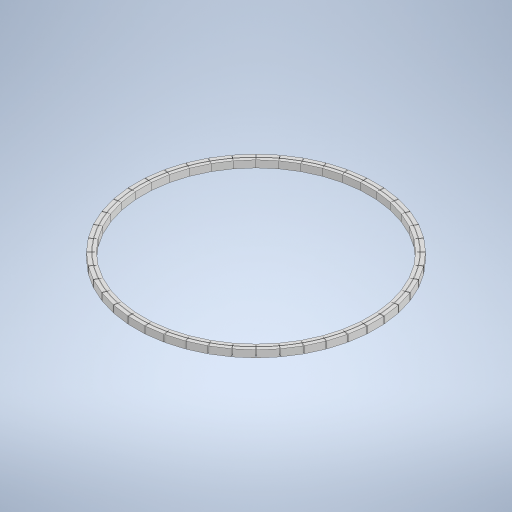
# Autodesk Inventor part: 柱-1 磚-1
Saved by Autodesk Inventor 2024 (Build 280153000, 153)
## iProperties
Created: 2024-05-18
Part Number: 柱-1 磚-1
Material: 一般
Document SubType Name: Modeling
Designer: User
Density: 1 g/cm^3
Appearance: 預設
Author: User
Autodesk Inventor part; units mm, degrees
ref_plane "YZ Plane" through (0, 0, 0) normal (1, 0, 0) x (0, 1, 0)
ref_plane "XZ Plane" through (0, 0, 0) normal (0, 1, 0) x (-1, 0, 0)
ref_plane "XY Plane" through (0, 0, 0) normal (0, 0, 1) x (1, 0, 0)
sketch "草圖1" plane through (0, 0, 0) normal (0, 1, 0) x (-1, 0, 0)
  circle A0 centre (0, 0) radius 25
  line L0 (24.25, 1.75) -> (25.75, 1.75)
  line L1 (25.75, 1.75) -> (25.75, -1.75)
  line L2 (25.75, -1.75) -> (24.25, -1.75)
  line L3 (24.25, -1.75) -> (24.25, 1.75)
  line L4 (24.25, 1.75) -> (25.75, -1.75) construction
  line L5 (25.75, 1.75) -> (24.25, -1.75) construction
  line L6 (25.2389, 5.3968) -> (25.737, 1.9324)
  line L7 (25.737, 1.9324) -> (24.2522, 1.7189)
  line L8 (24.2522, 1.7189) -> (23.7541, 5.1833)
  line L9 (23.7541, 5.1833) -> (25.2389, 5.3968)
  line L10 (24.2139, 8.9337) -> (25.2, 5.5755)
  line L11 (25.2, 5.5755) -> (23.7607, 5.1529)
  line L12 (23.7607, 5.1529) -> (22.7747, 8.5111)
  line L13 (22.7747, 8.5111) -> (24.2139, 8.9337)
  line L14 (22.696, 12.2888) -> (24.15, 9.1051)
  line L15 (24.15, 9.1051) -> (22.7856, 8.482)
  line L16 (22.7856, 8.482) -> (21.3316, 11.6657)
  line L17 (21.3316, 11.6657) -> (22.696, 12.2888)
  line L18 (20.7162, 15.3937) -> (22.6084, 12.4493)
  line L19 (22.6084, 12.4493) -> (21.3465, 11.6383)
  line L20 (21.3465, 11.6383) -> (19.4543, 14.5827)
  line L21 (19.4543, 14.5827) -> (20.7162, 15.3937)
  line L22 (18.3145, 18.1852) -> (20.6066, 15.5401)
  line L23 (20.6066, 15.5401) -> (19.4729, 14.5578)
  line L24 (19.4729, 14.5578) -> (17.1809, 17.2029)
  line L25 (17.1809, 17.2029) -> (18.3145, 18.1852)
  line L26 (15.5401, 20.6066) -> (18.1852, 18.3145)
  line L27 (18.1852, 18.3145) -> (17.2029, 17.1809)
  line L28 (17.2029, 17.1809) -> (14.5578, 19.4729)
  line L29 (14.5578, 19.4729) -> (15.5401, 20.6066)
  line L30 (12.4493, 22.6084) -> (15.3937, 20.7162)
  line L31 (15.3937, 20.7162) -> (14.5827, 19.4543)
  line L32 (14.5827, 19.4543) -> (11.6383, 21.3465)
  line L33 (11.6383, 21.3465) -> (12.4493, 22.6084)
  line L34 (9.1051, 24.15) -> (12.2888, 22.696)
  line L35 (12.2888, 22.696) -> (11.6657, 21.3316)
  line L36 (11.6657, 21.3316) -> (8.482, 22.7856)
  line L37 (8.482, 22.7856) -> (9.1051, 24.15)
  line L38 (5.5755, 25.2) -> (8.9337, 24.2139)
  line L39 (8.9337, 24.2139) -> (8.5111, 22.7747)
  line L40 (8.5111, 22.7747) -> (5.1529, 23.7607)
  line L41 (5.1529, 23.7607) -> (5.5755, 25.2)
  line L42 (1.9324, 25.737) -> (5.3968, 25.2389)
  line L43 (5.3968, 25.2389) -> (5.1833, 23.7541)
  line L44 (5.1833, 23.7541) -> (1.7189, 24.2522)
  line L45 (1.7189, 24.2522) -> (1.9324, 25.737)
  line L46 (-1.75, 25.75) -> (1.75, 25.75)
  line L47 (1.75, 25.75) -> (1.75, 24.25)
  line L48 (1.75, 24.25) -> (-1.75, 24.25)
  line L49 (-1.75, 24.25) -> (-1.75, 25.75)
  line L50 (-5.3968, 25.2389) -> (-1.9324, 25.737)
  line L51 (-1.9324, 25.737) -> (-1.7189, 24.2522)
  line L52 (-1.7189, 24.2522) -> (-5.1833, 23.7541)
  line L53 (-5.1833, 23.7541) -> (-5.3968, 25.2389)
  line L54 (-8.9337, 24.2139) -> (-5.5755, 25.2)
  line L55 (-5.5755, 25.2) -> (-5.1529, 23.7607)
  line L56 (-5.1529, 23.7607) -> (-8.5111, 22.7747)
  line L57 (-8.5111, 22.7747) -> (-8.9337, 24.2139)
  line L58 (-12.2888, 22.696) -> (-9.1051, 24.15)
  line L59 (-9.1051, 24.15) -> (-8.482, 22.7856)
  line L60 (-8.482, 22.7856) -> (-11.6657, 21.3316)
  line L61 (-11.6657, 21.3316) -> (-12.2888, 22.696)
  line L62 (-15.3937, 20.7162) -> (-12.4493, 22.6084)
  line L63 (-12.4493, 22.6084) -> (-11.6383, 21.3465)
  line L64 (-11.6383, 21.3465) -> (-14.5827, 19.4543)
  line L65 (-14.5827, 19.4543) -> (-15.3937, 20.7162)
  line L66 (-18.1852, 18.3145) -> (-15.5401, 20.6066)
  line L67 (-15.5401, 20.6066) -> (-14.5578, 19.4729)
  line L68 (-14.5578, 19.4729) -> (-17.2029, 17.1809)
  line L69 (-17.2029, 17.1809) -> (-18.1852, 18.3145)
  line L70 (-20.6066, 15.5401) -> (-18.3145, 18.1852)
  line L71 (-18.3145, 18.1852) -> (-17.1809, 17.2029)
  line L72 (-17.1809, 17.2029) -> (-19.4729, 14.5578)
  line L73 (-19.4729, 14.5578) -> (-20.6066, 15.5401)
  line L74 (-22.6084, 12.4493) -> (-20.7162, 15.3937)
  line L75 (-20.7162, 15.3937) -> (-19.4543, 14.5827)
  line L76 (-19.4543, 14.5827) -> (-21.3465, 11.6383)
  line L77 (-21.3465, 11.6383) -> (-22.6084, 12.4493)
  line L78 (-24.15, 9.1051) -> (-22.696, 12.2888)
  line L79 (-22.696, 12.2888) -> (-21.3316, 11.6657)
  line L80 (-21.3316, 11.6657) -> (-22.7856, 8.482)
  line L81 (-22.7856, 8.482) -> (-24.15, 9.1051)
  line L82 (-25.2, 5.5755) -> (-24.2139, 8.9337)
  line L83 (-24.2139, 8.9337) -> (-22.7747, 8.5111)
  line L84 (-22.7747, 8.5111) -> (-23.7607, 5.1529)
  line L85 (-23.7607, 5.1529) -> (-25.2, 5.5755)
  line L86 (-25.737, 1.9324) -> (-25.2389, 5.3968)
  line L87 (-25.2389, 5.3968) -> (-23.7541, 5.1833)
  line L88 (-23.7541, 5.1833) -> (-24.2522, 1.7189)
  line L89 (-24.2522, 1.7189) -> (-25.737, 1.9324)
  line L90 (-25.75, -1.75) -> (-25.75, 1.75)
  line L91 (-25.75, 1.75) -> (-24.25, 1.75)
  line L92 (-24.25, 1.75) -> (-24.25, -1.75)
  line L93 (-24.25, -1.75) -> (-25.75, -1.75)
  line L94 (-25.2389, -5.3968) -> (-25.737, -1.9324)
  line L95 (-25.737, -1.9324) -> (-24.2522, -1.7189)
  line L96 (-24.2522, -1.7189) -> (-23.7541, -5.1833)
  line L97 (-23.7541, -5.1833) -> (-25.2389, -5.3968)
  line L98 (-24.2139, -8.9337) -> (-25.2, -5.5755)
  line L99 (-25.2, -5.5755) -> (-23.7607, -5.1529)
  line L100 (-23.7607, -5.1529) -> (-22.7747, -8.5111)
  line L101 (-22.7747, -8.5111) -> (-24.2139, -8.9337)
  line L102 (-22.696, -12.2888) -> (-24.15, -9.1051)
  line L103 (-24.15, -9.1051) -> (-22.7856, -8.482)
  line L104 (-22.7856, -8.482) -> (-21.3316, -11.6657)
  line L105 (-21.3316, -11.6657) -> (-22.696, -12.2888)
  line L106 (-20.7162, -15.3937) -> (-22.6084, -12.4493)
  line L107 (-22.6084, -12.4493) -> (-21.3465, -11.6383)
  line L108 (-21.3465, -11.6383) -> (-19.4543, -14.5827)
  line L109 (-19.4543, -14.5827) -> (-20.7162, -15.3937)
  line L110 (-18.3145, -18.1852) -> (-20.6066, -15.5401)
  line L111 (-20.6066, -15.5401) -> (-19.4729, -14.5578)
  line L112 (-19.4729, -14.5578) -> (-17.1809, -17.2029)
  line L113 (-17.1809, -17.2029) -> (-18.3145, -18.1852)
  line L114 (-15.5401, -20.6066) -> (-18.1852, -18.3145)
  line L115 (-18.1852, -18.3145) -> (-17.2029, -17.1809)
  line L116 (-17.2029, -17.1809) -> (-14.5578, -19.4729)
  line L117 (-14.5578, -19.4729) -> (-15.5401, -20.6066)
  line L118 (-12.4493, -22.6084) -> (-15.3937, -20.7162)
  line L119 (-15.3937, -20.7162) -> (-14.5827, -19.4543)
  line L120 (-14.5827, -19.4543) -> (-11.6383, -21.3465)
  line L121 (-11.6383, -21.3465) -> (-12.4493, -22.6084)
  line L122 (-9.1051, -24.15) -> (-12.2888, -22.696)
  line L123 (-12.2888, -22.696) -> (-11.6657, -21.3316)
  line L124 (-11.6657, -21.3316) -> (-8.482, -22.7856)
  line L125 (-8.482, -22.7856) -> (-9.1051, -24.15)
  line L126 (-5.5755, -25.2) -> (-8.9337, -24.2139)
  line L127 (-8.9337, -24.2139) -> (-8.5111, -22.7747)
  line L128 (-8.5111, -22.7747) -> (-5.1529, -23.7607)
  line L129 (-5.1529, -23.7607) -> (-5.5755, -25.2)
  line L130 (-1.9324, -25.737) -> (-5.3968, -25.2389)
  line L131 (-5.3968, -25.2389) -> (-5.1833, -23.7541)
  line L132 (-5.1833, -23.7541) -> (-1.7189, -24.2522)
  line L133 (-1.7189, -24.2522) -> (-1.9324, -25.737)
  line L134 (1.75, -25.75) -> (-1.75, -25.75)
  line L135 (-1.75, -25.75) -> (-1.75, -24.25)
  line L136 (-1.75, -24.25) -> (1.75, -24.25)
  line L137 (1.75, -24.25) -> (1.75, -25.75)
  line L138 (5.3968, -25.2389) -> (1.9324, -25.737)
  line L139 (1.9324, -25.737) -> (1.7189, -24.2522)
  line L140 (1.7189, -24.2522) -> (5.1833, -23.7541)
  line L141 (5.1833, -23.7541) -> (5.3968, -25.2389)
  line L142 (8.9337, -24.2139) -> (5.5755, -25.2)
  line L143 (5.5755, -25.2) -> (5.1529, -23.7607)
  line L144 (5.1529, -23.7607) -> (8.5111, -22.7747)
  line L145 (8.5111, -22.7747) -> (8.9337, -24.2139)
  line L146 (12.2888, -22.696) -> (9.1051, -24.15)
  line L147 (9.1051, -24.15) -> (8.482, -22.7856)
  line L148 (8.482, -22.7856) -> (11.6657, -21.3316)
  line L149 (11.6657, -21.3316) -> (12.2888, -22.696)
  line L150 (15.3937, -20.7162) -> (12.4493, -22.6084)
  line L151 (12.4493, -22.6084) -> (11.6383, -21.3465)
  line L152 (11.6383, -21.3465) -> (14.5827, -19.4543)
  line L153 (14.5827, -19.4543) -> (15.3937, -20.7162)
  line L154 (18.1852, -18.3145) -> (15.5401, -20.6066)
  line L155 (15.5401, -20.6066) -> (14.5578, -19.4729)
  line L156 (14.5578, -19.4729) -> (17.2029, -17.1809)
  line L157 (17.2029, -17.1809) -> (18.1852, -18.3145)
  line L158 (20.6066, -15.5401) -> (18.3145, -18.1852)
  line L159 (18.3145, -18.1852) -> (17.1809, -17.2029)
  line L160 (17.1809, -17.2029) -> (19.4729, -14.5578)
  line L161 (19.4729, -14.5578) -> (20.6066, -15.5401)
  line L162 (22.6084, -12.4493) -> (20.7162, -15.3937)
  line L163 (20.7162, -15.3937) -> (19.4543, -14.5827)
  line L164 (19.4543, -14.5827) -> (21.3465, -11.6383)
  line L165 (21.3465, -11.6383) -> (22.6084, -12.4493)
  line L166 (24.15, -9.1051) -> (22.696, -12.2888)
  line L167 (22.696, -12.2888) -> (21.3316, -11.6657)
  line L168 (21.3316, -11.6657) -> (22.7856, -8.482)
  line L169 (22.7856, -8.482) -> (24.15, -9.1051)
  line L170 (25.2, -5.5755) -> (24.2139, -8.9337)
  line L171 (24.2139, -8.9337) -> (22.7747, -8.5111)
  line L172 (22.7747, -8.5111) -> (23.7607, -5.1529)
  line L173 (23.7607, -5.1529) -> (25.2, -5.5755)
  line L174 (25.737, -1.9324) -> (25.2389, -5.3968)
  line L175 (25.2389, -5.3968) -> (23.7541, -5.1833)
  line L176 (23.7541, -5.1833) -> (24.2522, -1.7189)
  line L177 (24.2522, -1.7189) -> (25.737, -1.9324)
  point P0 (25, 0)
  point P1 (24.4682, 1.75)
  point P2 (23.9701, 5.2144)
  point P3 (22.984, 8.5726)
  point P4 (21.5301, 11.7563)
  point P5 (19.6378, 14.7007)
  point P6 (17.3458, 17.3458)
  point P7 (14.7007, 19.6378)
  point P8 (11.7563, 21.5301)
  point P9 (8.5726, 22.984)
  point P10 (5.2144, 23.9701)
  point P11 (1.75, 24.4682)
  point P12 (-1.75, 24.4682)
  point P13 (-5.2144, 23.9701)
  point P14 (-8.5726, 22.984)
  point P15 (-11.7563, 21.5301)
  point P16 (-14.7007, 19.6378)
  point P17 (-17.3458, 17.3458)
  point P18 (-19.6378, 14.7007)
  point P19 (-21.5301, 11.7563)
  point P20 (-22.984, 8.5726)
  point P21 (-23.9701, 5.2144)
  point P22 (-24.4682, 1.75)
  point P23 (-24.4682, -1.75)
  point P24 (-23.9701, -5.2144)
  point P25 (-22.984, -8.5726)
  point P26 (-21.5301, -11.7563)
  point P27 (-19.6378, -14.7007)
  point P28 (-17.3458, -17.3458)
  point P29 (-14.7007, -19.6378)
  point P30 (-11.7563, -21.5301)
  point P31 (-8.5726, -22.984)
  point P32 (-5.2144, -23.9701)
  point P33 (-1.75, -24.4682)
  point P34 (1.75, -24.4682)
  point P35 (5.2144, -23.9701)
  point P36 (8.5726, -22.984)
  point P37 (11.7563, -21.5301)
  point P38 (14.7007, -19.6378)
  point P39 (17.3458, -17.3458)
  point P40 (19.6378, -14.7007)
  point P41 (21.5301, -11.7563)
  point P42 (22.984, -8.5726)
  point P43 (23.9701, -5.2144)
  point P44 (24.4682, -1.75)
  point P45 (24.25, 1.7344)
  point P46 (24.25, -1.7344)
  point P47 (23.7563, -5.1679)
  point P48 (22.7791, -8.4962)
  point P49 (21.3381, -11.6515)
  point P50 (19.4627, -14.5696)
  point P51 (17.1911, -17.1911)
  point P52 (14.5696, -19.4627)
  point P53 (11.6515, -21.3381)
  point P54 (8.4962, -22.7791)
  point P55 (5.1679, -23.7563)
  point P56 (1.7344, -24.25)
  point P57 (-1.7344, -24.25)
  point P58 (-5.1679, -23.7563)
  point P59 (-8.4962, -22.7791)
  point P60 (-11.6515, -21.3381)
  point P61 (-14.5696, -19.4627)
  point P62 (-17.1911, -17.1911)
  point P63 (-19.4627, -14.5696)
  point P64 (-21.3381, -11.6515)
  point P65 (-22.7791, -8.4962)
  point P66 (-23.7563, -5.1679)
  point P67 (-24.25, -1.7344)
  point P68 (-24.25, 1.7344)
  point P69 (-23.7563, 5.1679)
  point P70 (-22.7791, 8.4962)
  point P71 (-21.3381, 11.6515)
  point P72 (-19.4627, 14.5696)
  point P73 (-17.1911, 17.1911)
  point P74 (-14.5696, 19.4627)
  point P75 (-11.6515, 21.3381)
  point P76 (-8.4962, 22.7791)
  point P77 (-5.1679, 23.7563)
  point P78 (-1.7344, 24.25)
  point P79 (1.7344, 24.25)
  point P80 (5.1679, 23.7563)
  point P81 (8.4962, 22.7791)
  point P82 (11.6515, 21.3381)
  point P83 (14.5696, 19.4627)
  point P84 (17.1911, 17.1911)
  point P85 (19.4627, 14.5696)
  point P86 (21.3381, 11.6515)
  point P87 (22.7791, 8.4962)
  point P88 (23.7563, 5.1679)
  dimension "d0" = 50
  dimension "d1" = 1.5
  dimension "d2" = 3.5
  dimension "d5" = 360
  constraints: 356 end point, 2 midpoint, 2 parallel, 1 coincident, 1 horizontal, 1 horizontal alignment, 1 perpendicular, 355 other
  measures "d1" distance of L1.end L2.end
  measures "d2" distance of L0.end L1.end
extrude "擠出1" add sketch "草圖1" along normal blind 1.5 contours A0 L2 L177 L176 L3 L8 L7 L0 | A0 L0 L1 L2 | L7 L0 L3 L8 L12 L11 L9 A0 | A0 L9 L6 L7 | L7 L8 L3 L0 | L177 L174 L175 A0 | A0 L175 L173 L172 L176 L3 L2 L177 | L2 L3 L176 L177 | L11 L9 L8 L12 L16 L15 L13 A0 | A0 L13 L10 L11 | L11 L12 L8 L9 | L173 L170 L171 A0 | A0 L171 L169 L168 L172 L176 L175 L173 | L175 L176 L172 L173 | L15 L13 L12 L16 L20 L19 L17 A0 | A0 L17 L14 L15 | L15 L16 L12 L13 | L169 L166 L167 A0 | A0 L167 L165 L164 L168 L172 L171 L169 | L171 L172 L168 L169 | L20 L24 L23 L21 A0 L19 L17 L16 | L16 L17 L19 L20 | L168 L167 L165 A0 L163 L161 L160 L164 | L164 L165 L167 L168 | A0 L21 L18 L19 | L24 L28 L27 L25 A0 L23 L21 L20 | L20 L21 L23 L24 | L165 L162 L163 A0 | L164 L163 L161 A0 L159 L157 L156 L160 | L160 L161 L163 L164 | L28 L32 L31 L29 A0 L27 L25 L24 | L24 L25 L27 L28 | L160 L159 L157 A0 L155 L153 L152 L156 | L156 L157 L159 L160 | A0 L25 L22 L23 | L32 L36 L35 L33 A0 L31 L29 L28 | L28 L29 L31 L32 | L161 L158 L159 A0 | L156 L155 L153 A0 L151 L149 L148 L152 | L152 L153 L155 L156 | L36 L40 L39 L37 A0 L35 L33 L32 | L32 L33 L35 L36 | L152 L151 L149 A0 L147 L145 L144 L148 | L148 L149 L151 L152 | A0 L29 L26 L27 | L40 L44 L43 L41 A0 L39 L37 L36 | L36 L37 L39 L40 | L157 L154 L155 A0 | L148 L147 L145 A0 L143 L141 L140 L144 | L144 L145 L147 L148 | A0 L33 L30 L31 | L44 L48 L47 L45 A0 L43 L41 L40 | L40 L41 L43 L44 | L144 L143 L141 A0 L139 L137 L136 L140 | L140 L141 L143 L144 | L153 L150 L151 A0 | A0 L37 L34 L35 | L48 L52 L51 L49 A0 L47 L45 L44 | L44 L45 L47 L48 | L140 L139 L137 A0 L135 L133 L132 L136 | L136 L137 L139 L140 | L149 L146 L147 A0 | A0 L41 L38 L39 | L52 L56 L55 L53 A0 L51 L49 L48 | L48 L49 L51 L52 | L136 L135 L133 A0 L131 L129 L128 L132 | L132 L133 L135 L136 | L145 L142 L143 A0 | A0 L45 L42 L43 | L56 L60 L59 L57 A0 L55 L53 L52 | L52 L53 L55 L56 | L132 L131 L129 A0 L127 L125 L124 L128 | L128 L129 L131 L132 | L141 L138 L139 A0 | A0 L49 L46 L47 | L60 L64 L63 L61 A0 L59 L57 L56 | L56 L57 L59 L60 | L128 L127 L125 A0 L123 L121 L120 L124 | L124 L125 L127 L128 | L137 L134 L135 A0 | A0 L53 L50 L51 | L64 L68 L67 L65 A0 L63 L61 L60 | L60 L61 L63 L64 | L124 L123 L121 A0 L119 L117 L116 L120 | L120 L121 L123 L124 | L133 L130 L131 A0 | A0 L57 L54 L55 | L68 L72 L71 L69 A0 L67 L65 L64 | L64 L65 L67 L68 | L120 L119 L117 A0 L115 L113 L112 L116 | L116 L117 L119 L120 | L129 L126 L127 A0 | A0 L61 L58 L59 | L72 L76 L75 L73 A0 L71 L69 L68 | L68 L69 L71 L72 | L116 L115 L113 A0 L111 L109 L108 L112 | L112 L113 L115 L116 | L125 L122 L123 A0 | A0 L65 L62 L63 | L76 L80 L79 L77 A0 L75 L73 L72 | L72 L73 L75 L76 | L112 L111 L109 A0 L107 L105 L104 L108 | L108 L109 L111 L112 | L121 L118 L119 A0 | A0 L69 L66 L67 | L80 L84 L83 L81 A0 L79 L77 L76 | L76 L77 L79 L80 | L108 L107 L105 A0 L103 L101 L100 L104 | L104 L105 L107 L108 | L117 L114 L115 A0 | A0 L73 L70 L71 | L84 L88 L87 L85 A0 L83 L81 L80 | L80 L81 L83 L84 | L104 L103 L101 A0 L99 L97 L96 L100 | L100 L101 L103 L104 | L113 L110 L111 A0 | A0 L77 L74 L75 | L88 L92 L91 L89 A0 L87 L85 L84 | L84 L85 L87 L88 | L100 L99 L97 A0 L95 L93 L92 L96 | L96 L97 L99 L100 | L109 L106 L107 A0 | A0 L81 L78 L79 | L92 L96 L95 L93 A0 L91 L89 L88 | L88 L89 L91 L92 | L92 L93 L95 L96 | L105 L102 L103 A0 | A0 L85 L82 L83 | L101 L98 L99 A0 | A0 L89 L86 L87 | L97 L94 L95 A0 | A0 L93 L90 L91
sketch "草圖2" plane through (0, 0, 0) normal (0, 1, 0) x (-1, 0, 0)
  circle A0 centre (0, 0) radius 24.95
  circle A1 centre (0, 0) radius 25.05
  dimension "d9" = 49.9
  dimension "d10" = 50.1
  constraints: 2 centre point, 2 coincident
  measures "d9" diameter of A0
  measures "d10" diameter of A1
extrude "擠出2" add sketch "草圖2" along normal blind 1.5 separate body
